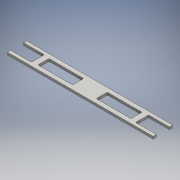
# Autodesk Inventor part: top
Saved by Autodesk Inventor 2016 (Build 200138000, 138)
## iProperties
Created: 2016-09-24
Part Number: top
Material: Generic
Document SubType Name: Modeling
Designer: Kevin G
Density: 1 g/cm^3
Appearance: Default
Author: Kevin G
Autodesk Inventor part; units mm, degrees
ref_plane "YZ Plane" through (0, 0, 0) normal (1, 0, 0) x (0, 1, 0)
ref_plane "XZ Plane" through (0, 0, 0) normal (0, 1, 0) x (-1, 0, 0)
ref_plane "XY Plane" through (0, 0, 0) normal (0, 0, 1) x (1, 0, 0)
sketch "Sketch1" plane through (0, 0, 0) normal (0, 0, 1) x (1, 0, 0)
  line L0 (282.4312, 43.9885) -> (-286.5277, 43.9885)
  line L1 (-286.5288, -32.1915) -> (282.4312, -32.1915)
  line L2 (-286.5277, 43.9885) -> (-286.5277, 31.2885)
  line L3 (-286.5288, -19.4915) -> (-286.5288, -32.1915)
  line L4 (282.4312, 31.3086) -> (282.4312, 43.9885)
  line L5 (282.4312, -19.4915) -> (282.4312, -32.1915)
  arc A0 (-205.7269, 29.0424) -> (-209.4741, 31.2885) centre (-209.4741, 27.0395) ccw
  arc A1 (-205.2441, 26.6389) -> (-205.7269, 29.0424) centre (-209.4741, 27.0395) ccw
  arc A2 (-209.4751, -19.4915) -> (-205.2441, -15.2625) centre (-209.4741, -15.2615) ccw
  arc A3 (-179.9924, 27.4418) -> (-183.6588, 23.2495) centre (-179.4288, 23.2495) ccw
  arc A4 (-183.6588, -11.4325) -> (-179.4288, -15.6625) centre (-179.4288, -11.4325) ccw
  arc A5 (-48.2006, 23.2495) -> (-52.4306, 27.4418) centre (-52.4304, 23.2118) ccw
  arc A6 (-52.9924, -15.6625) -> (-48.2006, -11.4325) centre (-52.4304, -11.47) ccw
  line L6 (-52.4306, 27.4418) -> (-179.9924, 27.4418)
  line L7 (-52.9924, -15.6625) -> (-179.4288, -15.6625)
  line L8 (-48.2006, -11.4325) -> (-48.2006, 23.2495)
  line L9 (-183.6588, -11.4325) -> (-183.6588, 23.2495)
  arc A7 (205.3642, 31.3086) -> (201.1322, 27.4399) centre (205.3642, 27.0596) ccw
  arc A8 (201.1322, -15.2425) -> (205.3812, -19.4915) centre (205.3812, -15.2425) ccw
  line L10 (201.1322, -15.2425) -> (201.1322, 23.2474)
  line L11 (201.1322, 23.2474) -> (201.1322, 27.4399)
  line L12 (282.4312, 31.3086) -> (205.3642, 31.3086)
  line L13 (282.4312, -19.4915) -> (205.3812, -19.4915)
  line L14 (-286.5288, -19.4915) -> (-209.4751, -19.4915)
  line L15 (-286.5277, 31.2885) -> (-209.4741, 31.2885)
  line L16 (-205.2441, 26.6389) -> (-205.2441, -15.2625)
  arc A9 (48.2152, 27.4415) -> (43.9852, 23.2115) centre (48.2152, 23.2115) ccw
  arc A10 (43.9852, -11.4145) -> (48.2152, -15.6445) centre (48.2152, -11.4145) ccw
  arc A11 (179.5472, 23.2115) -> (175.3172, 27.4415) centre (175.3172, 23.2115) ccw
  arc A12 (175.3172, -15.6445) -> (179.5472, -11.4145) centre (175.3172, -11.4145) ccw
  line L17 (48.2152, 27.4415) -> (175.3172, 27.4415)
  line L18 (48.2152, -15.6445) -> (175.3172, -15.6445)
  line L19 (43.9852, 23.2115) -> (43.9852, -11.4145)
  line L20 (179.5472, 23.2115) -> (179.5472, -11.4145)
  point P0 (0, 0)
  point P1 (0, 0)
  dimension "d0" = 135.4582
  dimension "d1" = 43.1043
  dimension "d2" = 16.5467
  dimension "d3" = 16.529
  dimension "d4" = 21.5853
  dimension "d5" = 92.1858
  constraints: 42 end point, 28 point on circle, 13 centre point, 9 vertical, 7 horizontal, 3 tangent, 1 collinear, 1 parallel
  measures "d0" distance between parallel lines of L8 L9
  measures "d1" distance between parallel lines of L7 L6
  measures "d2" distance between parallel lines of L0 L6
  measures "d3" distance between parallel lines of L1 L7
  measures "d4" distance between parallel lines of L9 L16
  measures "d5" distance between parallel lines of L19 L8
extrude "Extrusion1" add sketch "Sketch1" along normal blind 9.525
body "Solid1"
